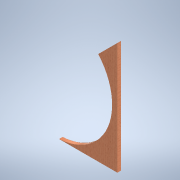
# Autodesk Inventor part: Hood (inside)
Saved by Autodesk Inventor 2020 (Build 240168000, 168)
## iProperties
Created: 2020-01-13
Part Number: Hood (inside)
Material: Wood (Oak)
Document SubType Name: Modeling
Designer: autum
Density: 0.76 g/cm^3
Appearance: White Oak - Natural Medium Gloss
Author: autum
Autodesk Inventor part; units mm, degrees
ref_plane "YZ Plane" through (0, 0, 0) normal (1, 0, 0) x (0, 1, 0)
ref_plane "XZ Plane" through (0, 0, 0) normal (0, 1, 0) x (-1, 0, 0)
ref_plane "XY Plane" through (0, 0, 0) normal (0, 0, 1) x (1, 0, 0)
sketch "Sketch1" plane through (0, 0, 0) normal (0, 0, 1) x (1, 0, 0)
  arc A0 (270.3829, -151.3678) -> (288.8718, 134.8752) centre (135.9788, 1.0322) ccw
  line L0 (358.2288, 204.2322) -> (358.2288, -202.1678)
  line L1 (358.2288, -202.1678) -> (147.3998, -202.1678)
  line L2 (147.3998, 204.2322) -> (553.7998, 204.2322) construction
  arc A1 (147.3998, -201.8466) -> (288.8718, 134.8752) centre (135.9788, 1.0322) ccw
  line L3 (147.3998, -201.8466) -> (147.3998, -202.1678)
  line L4 (358.2288, 204.2322) -> (288.8718, 134.8752)
  line L5 (358.2288, 204.2322) -> (456.3143, 204.2322) construction
  point P0 (270.3829, 153.4322)
  dimension "d5" = 203.2
  dimension "d9" = 135
  constraints: 12 end point, 4 point on circle, 2 centre point, 2 horizontal, 1 coincident, 1 equal length
  measures "d5" radius of A0
  measures "d9" angle of L4 L5
extrude "Extrusion1" add sketch "Sketch1" along normal blind 12.7
body "Solid1"
